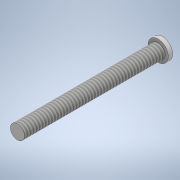
# Autodesk Inventor part: Screw
Saved by Autodesk Inventor 2020 (Build 240168000, 168)
## iProperties
Created: 2018-09-07
Part Number: Screw
Material: 일반
Document SubType Name: Modeling
Designer: Jeong Ji Hoon
Density: 1 g/cm^3
Appearance: 기본값
Author: Jeong Ji Hoon
Autodesk Inventor part; units mm, degrees
ref_plane "YZ Plane" through (0, 0, 0) normal (1, 0, 0) x (0, 1, 0)
ref_plane "XZ Plane" through (0, 0, 0) normal (0, 1, 0) x (-1, 0, 0)
ref_plane "XY Plane" through (0, 0, 0) normal (0, 0, 1) x (1, 0, 0)
sketch "스케치3" plane through (0, 0, 0) normal (0, 0, 1) x (1, 0, 0)
  line L0 (0, 0) -> (1.15, 0)
  line L1 (1.15, 0) -> (1.15, -0.5)
  line L2 (1.15, -0.5) -> (0.8, -0.5)
  line L3 (0.8, -0.5) -> (0.8, -16.5)
  line L4 (0.8, -16.5) -> (0, -16.5)
  line L5 (0, -16.5) -> (0, 0)
  dimension "d13" = 1.15
  dimension "d14" = 0.5
  dimension "d15" = 16
  dimension "d16" = 0.8
  constraints: 12 end point, 4 perpendicular, 1 horizontal, 1 parallel
  measures "d13" distance of L0.start L0.end
  measures "d14" distance of L0.end L1.end
  measures "d15" distance of L2.end L3.end
  measures "d16" distance of L3.end L4.end
revolve "회전2" add sketch "스케치3" angle 360 about axis through (0, -16.5, 0) along (0, 1, 0)
thread "스레드2" size "M1.6x0.35" class "6g" standard "ISO Metric profile" full length
sketch "스케치4" plane through (0, 0, 0) normal (0, 1, 0) x (1, 0, 0)
  line L0 (-0.15, -0.8) -> (0.15, -0.8)
  line L1 (0.15, -0.8) -> (0.15, 0.8)
  line L2 (0.15, 0.8) -> (-0.15, 0.8)
  line L3 (-0.15, 0.8) -> (-0.15, -0.8)
  line L4 (-0.15, -0.8) -> (0.15, 0.8) construction
  line L5 (0.15, -0.8) -> (-0.15, 0.8) construction
  line L6 (0.8, -0.15) -> (-0.8, -0.15)
  line L7 (-0.8, -0.15) -> (-0.8, 0.15)
  line L8 (-0.8, 0.15) -> (0.8, 0.15)
  line L9 (0.8, 0.15) -> (0.8, -0.15)
  circle A0 centre (0, 0) radius 0.8 projected
  line L10 (0.8, -0.15) -> (-0.8, 0.15) construction
  line L11 (-0.8, -0.15) -> (0.8, 0.15) construction
  dimension "d21" = 0.3
  dimension "d22" = 1.6
  dimension "d23" = 1.6
  dimension "d24" = 0.3
  constraints: 24 end point, 4 midpoint, 4 parallel, 2 horizontal, 2 perpendicular
  measures "d21" distance of L2.end L1.end
  measures "d22" distance of L1.end L0.end
  measures "d23" distance of L7.end L8.end
  measures "d24" distance of L6.end L7.end
extrude "돌출2" cut sketch "스케치4" against normal blind 0.3 contours L3 A0 L0 | A0 L1 L0 | A0 L3 L6 L1 | L6 A0 L8 L3 | L3 L8 L1 L6 | L6 L7 A0 | L1 L8 A0 L6 | A0 L9 L6 | L3 A0 L1 L8 | L7 L8 A0 | A0 L8 L9 | L3 L2 A0 | A0 L2 L1
body "Solid1"
